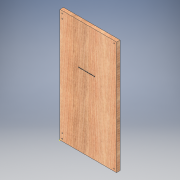
# Autodesk Inventor part: Middle Board
Saved by Autodesk Inventor 2018 (Build 220112000, 112)
## iProperties
Created: 2018-12-30
Part Number: Middle Board
Material: Generic
Document SubType Name: Modeling
Designer: maste
Density: 1 g/cm^3
Appearance: Default
Author: maste
Autodesk Inventor part; units mm, degrees
(part 1 of 2)
ref_plane "YZ Plane" through (0, 0, 0) normal (1, 0, 0) x (0, 1, 0)
ref_plane "XZ Plane" through (0, 0, 0) normal (0, 1, 0) x (-1, 0, 0)
ref_plane "XY Plane" through (0, 0, 0) normal (0, 0, 1) x (1, 0, 0)
sketch "Sketch1" plane through (0, 0, 0) normal (0, 0, 1) x (1, 0, 0)
  line L0 (0, 0) -> (304.8, 0)
  line L1 (304.8, 0) -> (304.8, 609.6)
  line L2 (304.8, 609.6) -> (0, 609.6)
  line L3 (0, 609.6) -> (0, 0)
  dimension "d0" = 304.8
  dimension "d1" = 609.6
  constraints: 8 end point, 2 parallel, 1 horizontal, 1 perpendicular
  measures "d0" distance of L2.end L1.end
  measures "d1" distance of L1.end L0.end
extrude "Extrusion1" add sketch "Sketch1" along normal blind 19.05
sketch "Sketch2" plane through (0, 0, 19.05) normal (0, 0, 1) x (1, 0, 0)
  line L0 (0, 0) -> (12.7, 0) construction
  line L1 (12.7, 0) -> (0, 0) construction
  line L2 (0, 0) -> (304.8, 0) construction
  line L3 (12.7, 0) -> (0, 0) construction
  line L4 (0, 0) -> (0, 12.7) construction
  line L5 (0, 609.6) -> (0, 0) construction
  line L6 (0, 12.7) -> (12.7, 12.7) construction
  circle A0 centre (12.7, 12.7) radius 2.5797
  line L7 (304.8, 0) -> (304.8, 609.6) construction
  line L8 (304.8, 304.8) -> (0, 304.8) construction
  line L9 (152.4, 0) -> (152.4, 609.6) construction
  line L10 (304.8, 609.6) -> (0, 609.6) construction
  circle A1 centre (12.7, 596.9) radius 2.5797
  circle A2 centre (292.1, 12.7) radius 2.5797
  circle A3 centre (292.1, 596.9) radius 2.5797
  line L11 (12.7, 596.9) -> (12.7, 571.5) construction
  circle A4 centre (12.7, 571.5) radius 2.5797
  circle A5 centre (12.7, 38.1) radius 2.5797
  dimension "d4" = 12.7
  dimension "d5" = 12.7
  dimension "d6" = 12.7
  dimension "d7" = 12.7
  dimension "d8" = 5.1594
  dimension "d11" = 25.4
  constraints: 16 end point, 6 centre point, 4 midpoint, 4 symmetric about line, 2 coincident, 1 collinear, 1 perpendicular, 1 point on line, 1 vertical, 4 other
  measures "d4" distance of L0.start L0.end
  measures "d5" distance of L0.end L0.start
  measures "d6" distance of L0.end L0.start
  measures "d7" distance of L0.start L4.end
  measures "d8" diameter of A0
  measures "d11" distance of L11.start L11.end
extrude "Extrusion3" cut sketch "Sketch2" against normal blind 19.05
sketch "Sketch3" plane through (0, 0, 19.05) normal (0, 0, 1) x (1, 0, 0)
  point P0 (0, 0)
sketch "Sketch4" plane through (0, 0, 0) normal (0, 0, -1) x (-1, 0, 0)
  line L0 (-188.1338, 391.5139) -> (-89.7519, 391.5139) construction
  line L1 (-89.7519, 391.5139) -> (-89.7519, 229.2701) construction
  line L2 (-89.7519, 229.2701) -> (-188.1338, 229.2701) construction
  line L3 (-188.1338, 229.2701) -> (-188.1338, 391.5139) construction
  spline S0 degree 2 poles (-185.9379, 389.5354) (-185.9379, 388.9624) (-186.4838, 388.2856) (-186.9012, 388.2856) knots 0 0 0 1 2 2 2
  spline S1 degree 2 poles (-186.9012, 388.2856) (-187.0717, 388.2856) (-187.3335, 388.3646) (-187.4694, 388.4461) knots 0 0 0 1 2 2 2
  line L4 (-187.4694, 388.4461) -> (-187.4694, 387.4878)
  line L5 (-187.4694, 387.4878) -> (-187.8547, 387.4878)
  line L6 (-187.8547, 387.4878) -> (-187.8547, 390.6173)
  line L7 (-187.8547, 390.6173) -> (-187.4694, 390.6173)
  line L8 (-187.4694, 390.6173) -> (-187.4694, 390.3777)
  spline S2 degree 2 poles (-187.4694, 390.3777) (-187.3261, 390.5086) (-186.9753, 390.6815) (-186.7703, 390.6815) knots 0 0 0 1 2 2 2
  spline S3 degree 2 poles (-186.7703, 390.6815) (-186.3776, 390.6815) (-185.9379, 390.0591) (-185.9379, 389.5354) knots 0 0 0 1 2 2 2
  spline S4 degree 2 poles (-186.3356, 389.491) (-186.3356, 389.8837) (-186.5851, 390.3159) (-186.8642, 390.3159) knots 0 0 0 1 2 2 2
  spline S5 degree 2 poles (-186.8642, 390.3159) (-187.0272, 390.3159) (-187.3335, 390.1702) (-187.4694, 390.0566) knots 0 0 0 1 2 2 2
  line L9 (-187.4694, 390.0566) -> (-187.4694, 388.7574)
  spline S6 degree 2 poles (-187.4694, 388.7574) (-187.3187, 388.6857) (-187.1038, 388.6314) (-186.9655, 388.6314) knots 0 0 0 1 2 2 2
  spline S7 degree 2 poles (-186.9655, 388.6314) (-186.6666, 388.6314) (-186.3356, 389.071) (-186.3356, 389.491) knots 0 0 0 1 2 2 2
  line L10 (-183.7594, 388.33) -> (-184.1447, 388.33)
  line L11 (-184.1447, 388.33) -> (-184.1447, 388.582)
  spline S8 degree 2 poles (-184.1447, 388.582) (-184.3226, 388.4264) (-184.6412, 388.2658) (-184.8388, 388.2658) knots 0 0 0 1 2 2 2
  spline S9 degree 2 poles (-184.8388, 388.2658) (-184.987, 388.2658) (-185.2513, 388.3646) (-185.3476, 388.4708) knots 0 0 0 1 2 2 2
  spline S10 degree 2 poles (-185.3476, 388.4708) (-185.4464, 388.577) (-185.5551, 388.9006) (-185.5551, 389.1328) knots 0 0 0 1 2 2 2
  line L12 (-185.5551, 389.1328) -> (-185.5551, 390.6173)
  line L13 (-185.5551, 390.6173) -> (-185.1698, 390.6173)
  line L14 (-185.1698, 390.6173) -> (-185.1698, 389.3131)
  spline S11 degree 2 poles (-185.1698, 389.3131) (-185.1698, 389.1303) (-185.1426, 388.8907) (-185.0957, 388.8018) knots 0 0 0 1 2 2 2
  spline S12 degree 2 poles (-185.0957, 388.8018) (-185.0487, 388.7129) (-184.8882, 388.6314) (-184.7375, 388.6314) knots 0 0 0 1 2 2 2
  spline S13 degree 2 poles (-184.7375, 388.6314) (-184.5967, 388.6314) (-184.2781, 388.7919) (-184.1447, 388.908) knots 0 0 0 1 2 2 2
  line L15 (-184.1447, 388.908) -> (-184.1447, 390.6173)
  line L16 (-184.1447, 390.6173) -> (-183.7594, 390.6173)
  line L17 (-183.7594, 390.6173) -> (-183.7594, 388.33)
  spline S14 degree 2 poles (-182.5096, 388.2856) (-182.8233, 388.2856) (-183.1765, 388.6437) (-183.1765, 389.0315) knots 0 0 0 1 2 2 2
  line L18 (-183.1765, 389.0315) -> (-183.1765, 390.2986)
  line L19 (-183.1765, 390.2986) -> (-183.4358, 390.2986)
  line L20 (-183.4358, 390.2986) -> (-183.4358, 390.6173)
  line L21 (-183.4358, 390.6173) -> (-183.1765, 390.6173)
  line L22 (-183.1765, 390.6173) -> (-183.1765, 391.2743)
  line L23 (-183.1765, 391.2743) -> (-182.7911, 391.2743)
  line L24 (-182.7911, 391.2743) -> (-182.7911, 390.6173)
  line L25 (-182.7911, 390.6173) -> (-182.0822, 390.6173)
  line L26 (-182.0822, 390.6173) -> (-182.0822, 390.2986)
  line L27 (-182.0822, 390.2986) -> (-182.7911, 390.2986)
  line L28 (-182.7911, 390.2986) -> (-182.7911, 389.2094)
  spline S15 degree 2 poles (-182.7911, 389.2094) (-182.7911, 389.0365) (-182.7788, 388.8463) (-182.7368, 388.7648) knots 0 0 0 1 2 2 2
  spline S16 degree 2 poles (-182.7368, 388.7648) (-182.7022, 388.6931) (-182.5466, 388.6215) (-182.4132, 388.6215) knots 0 0 0 1 2 2 2
  spline S17 degree 2 poles (-182.4132, 388.6215) (-182.3194, 388.6215) (-182.144, 388.6783) (-182.1045, 388.6956) knots 0 0 0 1 2 2 2
  line L29 (-182.1045, 388.6956) -> (-182.0822, 388.6956)
  line L30 (-182.0822, 388.6956) -> (-182.0822, 388.3498)
  spline S18 degree 2 poles (-182.0822, 388.3498) (-182.1909, 388.3202) (-182.4132, 388.2856) (-182.5096, 388.2856) knots 0 0 0 1 2 2 2
  spline S19 degree 2 poles (-179.8716, 388.2757) (-180.1013, 388.2757) (-180.499, 388.3992) (-180.6299, 388.4684) knots 0 0 0 1 2 2 2
  line L31 (-180.6299, 388.4684) -> (-180.6299, 388.9006)
  line L32 (-180.6299, 388.9006) -> (-180.6101, 388.9006)
  spline S20 degree 2 poles (-180.6101, 388.9006) (-180.5607, 388.8611) (-180.4273, 388.7672) (-180.3162, 388.7154) knots 0 0 0 1 2 2 2
  spline S21 degree 2 poles (-180.3162, 388.7154) (-180.2199, 388.6684) (-179.9827, 388.5993) (-179.8568, 388.5993) knots 0 0 0 1 2 2 2
  spline S22 degree 2 poles (-179.8568, 388.5993) (-179.7654, 388.5993) (-179.5554, 388.6413) (-179.506, 388.6758) knots 0 0 0 1 2 2 2
  spline S23 degree 2 poles (-179.506, 388.6758) (-179.4344, 388.7228) (-179.3702, 388.829) (-179.3702, 388.9377) knots 0 0 0 1 2 2 2
  spline S24 degree 2 poles (-179.3702, 388.9377) (-179.3702, 389.0735) (-179.5184, 389.2143) (-179.7086, 389.2612) knots 0 0 0 1 2 2 2
  spline S25 degree 2 poles (-179.7086, 389.2612) (-179.7827, 389.2785) (-180.0198, 389.3279) (-180.1211, 389.3551) knots 0 0 0 1 2 2 2
  spline S26 degree 2 poles (-180.1211, 389.3551) (-180.3829, 389.4317) (-180.62, 389.7478) (-180.62, 389.9726) knots 0 0 0 1 2 2 2
  spline S27 degree 2 poles (-180.62, 389.9726) (-180.62, 390.2838) (-180.1532, 390.6716) (-179.7678, 390.6716) knots 0 0 0 1 2 2 2
  spline S28 degree 2 poles (-179.7678, 390.6716) (-179.5777, 390.6716) (-179.1923, 390.5778) (-179.0614, 390.5061) knots 0 0 0 1 2 2 2
  line L33 (-179.0614, 390.5061) -> (-179.0614, 390.0936)
  line L34 (-179.0614, 390.0936) -> (-179.0812, 390.0936)
  spline S29 degree 2 poles (-179.0812, 390.0936) (-179.2294, 390.2122) (-179.59, 390.348) (-179.7753, 390.348) knots 0 0 0 1 2 2 2
  spline S30 degree 2 poles (-179.7753, 390.348) (-179.9654, 390.348) (-180.2273, 390.1875) (-180.2273, 390.0269) knots 0 0 0 1 2 2 2
  spline S31 degree 2 poles (-180.2273, 390.0269) (-180.2273, 389.8812) (-180.0717, 389.7404) (-179.8988, 389.696) knots 0 0 0 1 2 2 2
  spline S32 degree 2 poles (-179.8988, 389.696) (-179.8148, 389.6737) (-179.6024, 389.6293) (-179.4863, 389.6021) knots 0 0 0 1 2 2 2
  spline S33 degree 2 poles (-179.4863, 389.6021) (-179.2343, 389.5379) (-178.9774, 389.2439) (-178.9774, 388.9895) knots 0 0 0 1 2 2 2
  spline S34 degree 2 poles (-178.9774, 388.9895) (-178.9774, 388.8413) (-179.0935, 388.5795) (-179.2071, 388.4832) knots 0 0 0 1 2 2 2
  spline S35 degree 2 poles (-179.2071, 388.4832) (-179.3282, 388.3819) (-179.6369, 388.2757) (-179.8716, 388.2757) knots 0 0 0 1 2 2 2
  spline S36 degree 2 poles (-176.7396, 389.4737) (-176.7396, 388.8957) (-177.2954, 388.2658) (-177.7597, 388.2658) knots 0 0 0 1 2 2 2
  spline S37 degree 2 poles (-177.7597, 388.2658) (-178.2364, 388.2658) (-178.7823, 388.9154) (-178.7823, 389.4737) knots 0 0 0 1 2 2 2
  spline S38 degree 2 poles (-178.7823, 389.4737) (-178.7823, 390.0467) (-178.2191, 390.6815) (-177.7597, 390.6815) knots 0 0 0 1 2 2 2
  spline S39 degree 2 poles (-177.7597, 390.6815) (-177.2954, 390.6815) (-176.7396, 390.0492) (-176.7396, 389.4737) knots 0 0 0 1 2 2 2
  spline S40 degree 2 poles (-177.1373, 389.4737) (-177.1373, 389.9183) (-177.4608, 390.3505) (-177.7597, 390.3505) knots 0 0 0 1 2 2 2
  spline S41 degree 2 poles (-177.7597, 390.3505) (-178.0586, 390.3505) (-178.3846, 389.9183) (-178.3846, 389.4737) knots 0 0 0 1 2 2 2
  spline S42 degree 2 poles (-178.3846, 389.4737) (-178.3846, 389.0414) (-178.0586, 388.5968) (-177.7597, 388.5968) knots 0 0 0 1 2 2 2
  spline S43 degree 2 poles (-177.7597, 388.5968) (-177.4633, 388.5968) (-177.1373, 389.034) (-177.1373, 389.4737) knots 0 0 0 1 2 2 2
  line L35 (-173.7509, 388.33) -> (-173.7509, 389.654)
  spline S44 degree 2 poles (-173.7509, 389.654) (-173.7509, 389.8121) (-173.7756, 390.0813) (-173.8151, 390.1554) knots 0 0 0 1 2 2 2
  spline S45 degree 2 poles (-173.8151, 390.1554) (-173.8546, 390.2369) (-174.0053, 390.3159) (-174.1362, 390.3159) knots 0 0 0 1 2 2 2
  spline S46 degree 2 poles (-174.1362, 390.3159) (-174.2548, 390.3159) (-174.5265, 390.1702) (-174.6697, 390.0319) knots 0 0 0 1 2 2 2
  spline S47 degree 2 poles (-174.6697, 390.0319) (-174.6673, 389.9973) (-174.6623, 389.901) (-174.6623, 389.8368) knots 0 0 0 1 2 2 2
  line L36 (-174.6623, 389.8368) -> (-174.6623, 388.33)
  line L37 (-174.6623, 388.33) -> (-175.0476, 388.33)
  line L38 (-175.0476, 388.33) -> (-175.0476, 389.654)
  spline S48 degree 2 poles (-175.0476, 389.654) (-175.0476, 389.8121) (-175.0723, 390.0813) (-175.1119, 390.1554) knots 0 0 0 1 2 2 2
  spline S49 degree 2 poles (-175.1119, 390.1554) (-175.1514, 390.2369) (-175.3021, 390.3159) (-175.433, 390.3159) knots 0 0 0 1 2 2 2
  spline S50 degree 2 poles (-175.433, 390.3159) (-175.5565, 390.3159) (-175.8306, 390.1603) (-175.9591, 390.0393) knots 0 0 0 1 2 2 2
  line L39 (-175.9591, 390.0393) -> (-175.9591, 388.33)
  line L40 (-175.9591, 388.33) -> (-176.3444, 388.33)
  line L41 (-176.3444, 388.33) -> (-176.3444, 390.6173)
  line L42 (-176.3444, 390.6173) -> (-175.9591, 390.6173)
  line L43 (-175.9591, 390.6173) -> (-175.9591, 390.3653)
  spline S51 degree 2 poles (-175.9591, 390.3653) (-175.8084, 390.516) (-175.512, 390.6815) (-175.3342, 390.6815) knots 0 0 0 1 2 2 2
  spline S52 degree 2 poles (-175.3342, 390.6815) (-175.1316, 390.6815) (-174.8179, 390.4962) (-174.7364, 390.2863) knots 0 0 0 1 2 2 2
  spline S53 degree 2 poles (-174.7364, 390.2863) (-174.561, 390.4814) (-174.2301, 390.6815) (-174.0374, 390.6815) knots 0 0 0 1 2 2 2
  spline S54 degree 2 poles (-174.0374, 390.6815) (-173.8892, 390.6815) (-173.6471, 390.5901) (-173.5582, 390.4864) knots 0 0 0 1 2 2 2
  spline S55 degree 2 poles (-173.5582, 390.4864) (-173.4668, 390.3826) (-173.3656, 390.0714) (-173.3656, 389.8368) knots 0 0 0 1 2 2 2
  line L44 (-173.3656, 389.8368) -> (-173.3656, 388.33)
  line L45 (-173.3656, 388.33) -> (-173.7509, 388.33)
  spline S56 degree 2 poles (-171.8317, 388.2782) (-172.38, 388.2782) (-172.9827, 388.8932) (-172.9827, 389.4613) knots 0 0 0 1 2 2 2
  spline S57 degree 2 poles (-172.9827, 389.4613) (-172.9827, 390.0195) (-172.3973, 390.6815) (-171.9255, 390.6815) knots 0 0 0 1 2 2 2
  spline S58 degree 2 poles (-171.9255, 390.6815) (-171.7131, 390.6815) (-171.3846, 390.558) (-171.2636, 390.4271) knots 0 0 0 1 2 2 2
  spline S59 degree 2 poles (-171.2636, 390.4271) (-171.1401, 390.2962) (-171.0092, 389.9183) (-171.0092, 389.6441) knots 0 0 0 1 2 2 2
  line L46 (-171.0092, 389.6441) -> (-171.0092, 389.4341)
  line L47 (-171.0092, 389.4341) -> (-172.5924, 389.4341)
  spline S60 degree 2 poles (-172.5924, 389.4341) (-172.5924, 389.0365) (-172.1923, 388.6141) (-171.8366, 388.6141) knots 0 0 0 1 2 2 2
  spline S61 degree 2 poles (-171.8366, 388.6141) (-171.7106, 388.6141) (-171.4661, 388.6709) (-171.3673, 388.7154) knots 0 0 0 1 2 2 2
  spline S62 degree 2 poles (-171.3673, 388.7154) (-171.2636, 388.7648) (-171.1203, 388.8512) (-171.0734, 388.8907) knots 0 0 0 1 2 2 2
  line L48 (-171.0734, 388.8907) -> (-171.0512, 388.8907)
  line L49 (-171.0512, 388.8907) -> (-171.0512, 388.4708)
  spline S63 degree 2 poles (-171.0512, 388.4708) (-171.1178, 388.4437) (-171.3204, 388.3646) (-171.3994, 388.3424) knots 0 0 0 1 2 2 2
  spline S64 degree 2 poles (-171.3994, 388.3424) (-171.5106, 388.3103) (-171.6934, 388.2782) (-171.8317, 388.2782) knots 0 0 0 1 2 2 2
  spline S65 degree 2 poles (-171.3846, 389.7281) (-171.3895, 389.8837) (-171.4538, 390.1109) (-171.5155, 390.1875) knots 0 0 0 1 2 2 2
  spline S66 degree 2 poles (-171.5155, 390.1875) (-171.5822, 390.2739) (-171.7922, 390.3653) (-171.9478, 390.3653) knots 0 0 0 1 2 2 2
  spline S67 degree 2 poles (-171.9478, 390.3653) (-172.1009, 390.3653) (-172.3158, 390.2739) (-172.4047, 390.185) knots 0 0 0 1 2 2 2
  spline S68 degree 2 poles (-172.4047, 390.185) (-172.4912, 390.0936) (-172.5801, 389.8738) (-172.5924, 389.7281) knots 0 0 0 1 2 2 2
  line L50 (-172.5924, 389.7281) -> (-171.3846, 389.7281)
  line L51 (-168.9171, 388.33) -> (-169.3024, 388.33)
  line L52 (-169.3024, 388.33) -> (-169.3024, 391.5139)
  line L53 (-169.3024, 391.5139) -> (-168.9171, 391.5139)
  line L54 (-168.9171, 391.5139) -> (-168.9171, 388.33)
  spline S69 degree 2 poles (-167.0769, 388.5721) (-167.1238, 388.5375) (-167.2819, 388.414) (-167.356, 388.377) knots 0 0 0 1 2 2 2
  spline S70 degree 2 poles (-167.356, 388.377) (-167.4573, 388.3226) (-167.6475, 388.2658) (-167.8204, 388.2658) knots 0 0 0 1 2 2 2
  spline S71 degree 2 poles (-167.8204, 388.2658) (-167.9612, 388.2658) (-168.2156, 388.372) (-168.3119, 388.4684) knots 0 0 0 1 2 2 2
  spline S72 degree 2 poles (-168.3119, 388.4684) (-168.4033, 388.5622) (-168.5144, 388.8389) (-168.5144, 388.992) knots 0 0 0 1 2 2 2
  spline S73 degree 2 poles (-168.5144, 388.992) (-168.5144, 389.2291) (-168.3144, 389.5651) (-168.097, 389.6614) knots 0 0 0 1 2 2 2
  spline S74 degree 2 poles (-168.097, 389.6614) (-167.9044, 389.7503) (-167.3807, 389.817) (-167.0769, 389.8343) knots 0 0 0 1 2 2 2
  line L55 (-167.0769, 389.8343) -> (-167.0769, 389.9084)
  spline S75 degree 2 poles (-167.0769, 389.9084) (-167.0769, 390.0418) (-167.1584, 390.2073) (-167.2325, 390.2542) knots 0 0 0 1 2 2 2
  spline S76 degree 2 poles (-167.2325, 390.2542) (-167.3066, 390.3011) (-167.519, 390.3308) (-167.6327, 390.3308) knots 0 0 0 1 2 2 2
  spline S77 degree 2 poles (-167.6327, 390.3308) (-167.766, 390.3308) (-168.1267, 390.2517) (-168.307, 390.1751) knots 0 0 0 1 2 2 2
  line L56 (-168.307, 390.1751) -> (-168.3292, 390.1751)
  line L57 (-168.3292, 390.1751) -> (-168.3292, 390.5679)
  spline S78 degree 2 poles (-168.3292, 390.5679) (-168.223, 390.5975) (-167.8253, 390.6716) (-167.6302, 390.6716) knots 0 0 0 1 2 2 2
  spline S79 degree 2 poles (-167.6302, 390.6716) (-167.3931, 390.6716) (-167.0695, 390.5975) (-166.941, 390.5012) knots 0 0 0 1 2 2 2
  spline S80 degree 2 poles (-166.941, 390.5012) (-166.8151, 390.4073) (-166.6916, 390.1085) (-166.6916, 389.8936) knots 0 0 0 1 2 2 2
  line L58 (-166.6916, 389.8936) -> (-166.6916, 388.33)
  line L59 (-166.6916, 388.33) -> (-167.0769, 388.33)
  line L60 (-167.0769, 388.33) -> (-167.0769, 388.5721)
  line L61 (-167.0769, 388.8932) -> (-167.0769, 389.528)
  spline S81 degree 2 poles (-167.0769, 389.528) (-167.2152, 389.5157) (-167.6327, 389.4737) (-167.7636, 389.4341) knots 0 0 0 1 2 2 2
  spline S82 degree 2 poles (-167.7636, 389.4341) (-167.9167, 389.3872) (-168.1168, 389.1921) (-168.1168, 389.0192) knots 0 0 0 1 2 2 2
  spline S83 degree 2 poles (-168.1168, 389.0192) (-168.1168, 388.8216) (-167.8945, 388.6215) (-167.6821, 388.6215) knots 0 0 0 1 2 2 2
  spline S84 degree 2 poles (-167.6821, 388.6215) (-167.5017, 388.6215) (-167.2053, 388.7771) (-167.0769, 388.8932) knots 0 0 0 1 2 2 2
  spline S85 degree 2 poles (-164.2339, 389.5354) (-164.2339, 388.9624) (-164.7798, 388.2856) (-165.1972, 388.2856) knots 0 0 0 1 2 2 2
  spline S86 degree 2 poles (-165.1972, 388.2856) (-165.3676, 388.2856) (-165.6295, 388.3646) (-165.7653, 388.4461) knots 0 0 0 1 2 2 2
  line L62 (-165.7653, 388.4461) -> (-165.7653, 387.4878)
  line L63 (-165.7653, 387.4878) -> (-166.1506, 387.4878)
  line L64 (-166.1506, 387.4878) -> (-166.1506, 390.6173)
  line L65 (-166.1506, 390.6173) -> (-165.7653, 390.6173)
  line L66 (-165.7653, 390.6173) -> (-165.7653, 390.3777)
  spline S87 degree 2 poles (-165.7653, 390.3777) (-165.6221, 390.5086) (-165.2713, 390.6815) (-165.0663, 390.6815) knots 0 0 0 1 2 2 2
  spline S88 degree 2 poles (-165.0663, 390.6815) (-164.6736, 390.6815) (-164.2339, 390.0591) (-164.2339, 389.5354) knots 0 0 0 1 2 2 2
  spline S89 degree 2 poles (-164.6316, 389.491) (-164.6316, 389.8837) (-164.8811, 390.3159) (-165.1602, 390.3159) knots 0 0 0 1 2 2 2
  spline S90 degree 2 poles (-165.1602, 390.3159) (-165.3232, 390.3159) (-165.6295, 390.1702) (-165.7653, 390.0566) knots 0 0 0 1 2 2 2
  line L67 (-165.7653, 390.0566) -> (-165.7653, 388.7574)
  spline S91 degree 2 poles (-165.7653, 388.7574) (-165.6146, 388.6857) (-165.3998, 388.6314) (-165.2614, 388.6314) knots 0 0 0 1 2 2 2
  spline S92 degree 2 poles (-165.2614, 388.6314) (-164.9626, 388.6314) (-164.6316, 389.071) (-164.6316, 389.491) knots 0 0 0 1 2 2 2
  spline S93 degree 2 poles (-163.1422, 388.2856) (-163.4559, 388.2856) (-163.8091, 388.6437) (-163.8091, 389.0315) knots 0 0 0 1 2 2 2
  line L68 (-163.8091, 389.0315) -> (-163.8091, 390.2986)
  line L69 (-163.8091, 390.2986) -> (-164.0684, 390.2986)
  line L70 (-164.0684, 390.2986) -> (-164.0684, 390.6173)
  line L71 (-164.0684, 390.6173) -> (-163.8091, 390.6173)
  line L72 (-163.8091, 390.6173) -> (-163.8091, 391.2743)
  line L73 (-163.8091, 391.2743) -> (-163.4237, 391.2743)
  line L74 (-163.4237, 391.2743) -> (-163.4237, 390.6173)
  line L75 (-163.4237, 390.6173) -> (-162.7149, 390.6173)
  line L76 (-162.7149, 390.6173) -> (-162.7149, 390.2986)
  line L77 (-162.7149, 390.2986) -> (-163.4237, 390.2986)
  line L78 (-163.4237, 390.2986) -> (-163.4237, 389.2094)
  spline S94 degree 2 poles (-163.4237, 389.2094) (-163.4237, 389.0365) (-163.4114, 388.8463) (-163.3694, 388.7648) knots 0 0 0 1 2 2 2
  spline S95 degree 2 poles (-163.3694, 388.7648) (-163.3348, 388.6931) (-163.1792, 388.6215) (-163.0458, 388.6215) knots 0 0 0 1 2 2 2
  spline S96 degree 2 poles (-163.0458, 388.6215) (-162.952, 388.6215) (-162.7766, 388.6783) (-162.7371, 388.6956) knots 0 0 0 1 2 2 2
  line L79 (-162.7371, 388.6956) -> (-162.7149, 388.6956)
  line L80 (-162.7149, 388.6956) -> (-162.7149, 388.3498)
  spline S97 degree 2 poles (-162.7149, 388.3498) (-162.8235, 388.3202) (-163.0458, 388.2856) (-163.1422, 388.2856) knots 0 0 0 1 2 2 2
  spline S98 degree 2 poles (-160.5511, 389.4737) (-160.5511, 388.8957) (-161.1069, 388.2658) (-161.5712, 388.2658) knots 0 0 0 1 2 2 2
  spline S99 degree 2 poles (-161.5712, 388.2658) (-162.0479, 388.2658) (-162.5938, 388.9154) (-162.5938, 389.4737) knots 0 0 0 1 2 2 2
  spline S100 degree 2 poles (-162.5938, 389.4737) (-162.5938, 390.0467) (-162.0307, 390.6815) (-161.5712, 390.6815) knots 0 0 0 1 2 2 2
  spline S101 degree 2 poles (-161.5712, 390.6815) (-161.1069, 390.6815) (-160.5511, 390.0492) (-160.5511, 389.4737) knots 0 0 0 1 2 2 2
  spline S102 degree 2 poles (-160.9488, 389.4737) (-160.9488, 389.9183) (-161.2724, 390.3505) (-161.5712, 390.3505) knots 0 0 0 1 2 2 2
  spline S103 degree 2 poles (-161.5712, 390.3505) (-161.8701, 390.3505) (-162.1961, 389.9183) (-162.1961, 389.4737) knots 0 0 0 1 2 2 2
  spline S104 degree 2 poles (-162.1961, 389.4737) (-162.1961, 389.0414) (-161.8701, 388.5968) (-161.5712, 388.5968) knots 0 0 0 1 2 2 2
  spline S105 degree 2 poles (-161.5712, 388.5968) (-161.2748, 388.5968) (-160.9488, 389.034) (-160.9488, 389.4737) knots 0 0 0 1 2 2 2
  spline S106 degree 2 poles (-158.2392, 389.5354) (-158.2392, 388.9624) (-158.7851, 388.2856) (-159.2025, 388.2856) knots 0 0 0 1 2 2 2
  spline S107 degree 2 poles (-159.2025, 388.2856) (-159.3729, 388.2856) (-159.6347, 388.3646) (-159.7706, 388.4461) knots 0 0 0 1 2 2 2
  line L81 (-159.7706, 388.4461) -> (-159.7706, 387.4878)
  line L82 (-159.7706, 387.4878) -> (-160.1559, 387.4878)
  line L83 (-160.1559, 387.4878) -> (-160.1559, 390.6173)
  line L84 (-160.1559, 390.6173) -> (-159.7706, 390.6173)
  line L85 (-159.7706, 390.6173) -> (-159.7706, 390.3777)
  spline S108 degree 2 poles (-159.7706, 390.3777) (-159.6273, 390.5086) (-159.2766, 390.6815) (-159.0716, 390.6815) knots 0 0 0 1 2 2 2
  spline S109 degree 2 poles (-159.0716, 390.6815) (-158.6788, 390.6815) (-158.2392, 390.0591) (-158.2392, 389.5354) knots 0 0 0 1 2 2 2
  spline S110 degree 2 poles (-158.6369, 389.491) (-158.6369, 389.8837) (-158.8863, 390.3159) (-159.1654, 390.3159) knots 0 0 0 1 2 2 2
  spline S111 degree 2 poles (-159.1654, 390.3159) (-159.3285, 390.3159) (-159.6347, 390.1702) (-159.7706, 390.0566) knots 0 0 0 1 2 2 2
  line L86 (-159.7706, 390.0566) -> (-159.7706, 388.7574)
  spline S112 degree 2 poles (-159.7706, 388.7574) (-159.6199, 388.6857) (-159.405, 388.6314) (-159.2667, 388.6314) knots 0 0 0 1 2 2 2
  spline S113 degree 2 poles (-159.2667, 388.6314) (-158.9678, 388.6314) (-158.6369, 389.071) (-158.6369, 389.491) knots 0 0 0 1 2 2 2
  spline S114 degree 2 poles (-157.2215, 388.2757) (-157.4512, 388.2757) (-157.8489, 388.3992) (-157.9798, 388.4684) knots 0 0 0 1 2 2 2
  line L87 (-157.9798, 388.4684) -> (-157.9798, 388.9006)
  line L88 (-157.9798, 388.9006) -> (-157.9601, 388.9006)
  spline S115 degree 2 poles (-157.9601, 388.9006) (-157.9107, 388.8611) (-157.7773, 388.7672) (-157.6661, 388.7154) knots 0 0 0 1 2 2 2
  spline S116 degree 2 poles (-157.6661, 388.7154) (-157.5698, 388.6684) (-157.3327, 388.5993) (-157.2067, 388.5993) knots 0 0 0 1 2 2 2
  spline S117 degree 2 poles (-157.2067, 388.5993) (-157.1153, 388.5993) (-156.9054, 388.6413) (-156.856, 388.6758) knots 0 0 0 1 2 2 2
  spline S118 degree 2 poles (-156.856, 388.6758) (-156.7843, 388.7228) (-156.7201, 388.829) (-156.7201, 388.9377) knots 0 0 0 1 2 2 2
  spline S119 degree 2 poles (-156.7201, 388.9377) (-156.7201, 389.0735) (-156.8683, 389.2143) (-157.0585, 389.2612) knots 0 0 0 1 2 2 2
  spline S120 degree 2 poles (-157.0585, 389.2612) (-157.1326, 389.2785) (-157.3697, 389.3279) (-157.471, 389.3551) knots 0 0 0 1 2 2 2
  spline S121 degree 2 poles (-157.471, 389.3551) (-157.7328, 389.4317) (-157.9699, 389.7478) (-157.9699, 389.9726) knots 0 0 0 1 2 2 2
  spline S122 degree 2 poles (-157.9699, 389.9726) (-157.9699, 390.2838) (-157.5031, 390.6716) (-157.1178, 390.6716) knots 0 0 0 1 2 2 2
  spline S123 degree 2 poles (-157.1178, 390.6716) (-156.9276, 390.6716) (-156.5423, 390.5778) (-156.4114, 390.5061) knots 0 0 0 1 2 2 2
  line L89 (-156.4114, 390.5061) -> (-156.4114, 390.0936)
  line L90 (-156.4114, 390.0936) -> (-156.4311, 390.0936)
  spline S124 degree 2 poles (-156.4311, 390.0936) (-156.5793, 390.2122) (-156.94, 390.348) (-157.1252, 390.348) knots 0 0 0 1 2 2 2
  spline S125 degree 2 poles (-157.1252, 390.348) (-157.3154, 390.348) (-157.5772, 390.1875) (-157.5772, 390.0269) knots 0 0 0 1 2 2 2
  spline S126 degree 2 poles (-157.5772, 390.0269) (-157.5772, 389.8812) (-157.4216, 389.7404) (-157.2487, 389.696) knots 0 0 0 1 2 2 2
  spline S127 degree 2 poles (-157.2487, 389.696) (-157.1647, 389.6737) (-156.9523, 389.6293) (-156.8362, 389.6021) knots 0 0 0 1 2 2 2
  spline S128 degree 2 poles (-156.8362, 389.6021) (-156.5843, 389.5379) (-156.3274, 389.2439) (-156.3274, 388.9895) knots 0 0 0 1 2 2 2
  spline S129 degree 2 poles (-156.3274, 388.9895) (-156.3274, 388.8413) (-156.4435, 388.5795) (-156.5571, 388.4832) knots 0 0 0 1 2 2 2
  spline S130 degree 2 poles (-156.5571, 388.4832) (-156.6781, 388.3819) (-156.9869, 388.2757) (-157.2215, 388.2757) knots 0 0 0 1 2 2 2
  spline S131 degree 2 poles (-153.3856, 388.5721) (-153.4325, 388.5375) (-153.5906, 388.414) (-153.6647, 388.377) knots 0 0 0 1 2 2 2
  spline S132 degree 2 poles (-153.6647, 388.377) (-153.766, 388.3226) (-153.9562, 388.2658) (-154.1291, 388.2658) knots 0 0 0 1 2 2 2
  spline S133 degree 2 poles (-154.1291, 388.2658) (-154.2699, 388.2658) (-154.5243, 388.372) (-154.6206, 388.4684) knots 0 0 0 1 2 2 2
  spline S134 degree 2 poles (-154.6206, 388.4684) (-154.712, 388.5622) (-154.8231, 388.8389) (-154.8231, 388.992) knots 0 0 0 1 2 2 2
  spline S135 degree 2 poles (-154.8231, 388.992) (-154.8231, 389.2291) (-154.6231, 389.5651) (-154.4057, 389.6614) knots 0 0 0 1 2 2 2
  spline S136 degree 2 poles (-154.4057, 389.6614) (-154.2131, 389.7503) (-153.6894, 389.817) (-153.3856, 389.8343) knots 0 0 0 1 2 2 2
  line L91 (-153.3856, 389.8343) -> (-153.3856, 389.9084)
  spline S137 degree 2 poles (-153.3856, 389.9084) (-153.3856, 390.0418) (-153.4671, 390.2073) (-153.5412, 390.2542) knots 0 0 0 1 2 2 2
  spline S138 degree 2 poles (-153.5412, 390.2542) (-153.6153, 390.3011) (-153.8277, 390.3308) (-153.9414, 390.3308) knots 0 0 0 1 2 2 2
  spline S139 degree 2 poles (-153.9414, 390.3308) (-154.0747, 390.3308) (-154.4354, 390.2517) (-154.6157, 390.1751) knots 0 0 0 1 2 2 2
  line L92 (-154.6157, 390.1751) -> (-154.6379, 390.1751)
  line L93 (-154.6379, 390.1751) -> (-154.6379, 390.5679)
  spline S140 degree 2 poles (-154.6379, 390.5679) (-154.5317, 390.5975) (-154.134, 390.6716) (-153.9389, 390.6716) knots 0 0 0 1 2 2 2
  spline S141 degree 2 poles (-153.9389, 390.6716) (-153.7018, 390.6716) (-153.3782, 390.5975) (-153.2497, 390.5012) knots 0 0 0 1 2 2 2
  spline S142 degree 2 poles (-153.2497, 390.5012) (-153.1238, 390.4073) (-153.0003, 390.1085) (-153.0003, 389.8936) knots 0 0 0 1 2 2 2
  line L94 (-153.0003, 389.8936) -> (-153.0003, 388.33)
  line L95 (-153.0003, 388.33) -> (-153.3856, 388.33)
  line L96 (-153.3856, 388.33) -> (-153.3856, 388.5721)
  line L97 (-153.3856, 388.8932) -> (-153.3856, 389.528)
  spline S143 degree 2 poles (-153.3856, 389.528) (-153.5239, 389.5157) (-153.9414, 389.4737) (-154.0723, 389.4341) knots 0 0 0 1 2 2 2
  spline S144 degree 2 poles (-154.0723, 389.4341) (-154.2254, 389.3872) (-154.4255, 389.1921) (-154.4255, 389.0192) knots 0 0 0 1 2 2 2
  spline S145 degree 2 poles (-154.4255, 389.0192) (-154.4255, 388.8216) (-154.2032, 388.6215) (-153.9908, 388.6215) knots 0 0 0 1 2 2 2
  spline S146 degree 2 poles (-153.9908, 388.6215) (-153.8104, 388.6215) (-153.514, 388.7771) (-153.3856, 388.8932) knots 0 0 0 1 2 2 2
  line L98 (-150.6636, 388.33) -> (-151.049, 388.33)
  line L99 (-151.049, 388.33) -> (-151.049, 389.6342)
  spline S147 degree 2 poles (-151.049, 389.6342) (-151.049, 389.7923) (-151.0786, 390.064) (-151.1231, 390.1455) knots 0 0 0 1 2 2 2
  spline S148 degree 2 poles (-151.1231, 390.1455) (-151.17, 390.232) (-151.338, 390.3159) (-151.4812, 390.3159) knots 0 0 0 1 2 2 2
  spline S149 degree 2 poles (-151.4812, 390.3159) (-151.6245, 390.3159) (-151.9283, 390.1628) (-152.074, 390.0393) knots 0 0 0 1 2 2 2
  line L100 (-152.074, 390.0393) -> (-152.074, 388.33)
  line L101 (-152.074, 388.33) -> (-152.4593, 388.33)
  line L102 (-152.4593, 388.33) -> (-152.4593, 390.6173)
  line L103 (-152.4593, 390.6173) -> (-152.074, 390.6173)
  line L104 (-152.074, 390.6173) -> (-152.074, 390.3629)
  spline S150 degree 2 poles (-152.074, 390.3629) (-151.9011, 390.5185) (-151.5677, 390.6815) (-151.3799, 390.6815) knots 0 0 0 1 2 2 2
  spline S151 degree 2 poles (-151.3799, 390.6815) (-151.044, 390.6815) (-150.6636, 390.2369) (-150.6636, 389.8145) knots 0 0 0 1 2 2 2
  line L105 (-150.6636, 389.8145) -> (-150.6636, 388.33)
  line L106 (-148.3641, 388.33) -> (-148.7494, 388.33)
  line L107 (-148.7494, 388.33) -> (-148.7494, 388.5622)
  spline S152 degree 2 poles (-148.7494, 388.5622) (-148.8383, 388.4881) (-148.9692, 388.3893) (-149.0581, 388.3473) knots 0 0 0 1 2 2 2
  spline S153 degree 2 poles (-149.0581, 388.3473) (-149.1396, 388.3078) (-149.315, 388.2658) (-149.4311, 388.2658) knots 0 0 0 1 2 2 2
  spline S154 degree 2 poles (-149.4311, 388.2658) (-149.6188, 388.2658) (-149.935, 388.4214) (-150.0461, 388.5721) knots 0 0 0 1 2 2 2
  spline S155 degree 2 poles (-150.0461, 388.5721) (-150.1573, 388.7228) (-150.2808, 389.1674) (-150.2808, 389.4564) knots 0 0 0 1 2 2 2
  spline S156 degree 2 poles (-150.2808, 389.4564) (-150.2808, 389.7577) (-150.1252, 390.1974) (-149.9893, 390.3629) knots 0 0 0 1 2 2 2
  spline S157 degree 2 poles (-149.9893, 390.3629) (-149.8634, 390.5111) (-149.5101, 390.6815) (-149.315, 390.6815) knots 0 0 0 1 2 2 2
  spline S158 degree 2 poles (-149.315, 390.6815) (-149.1446, 390.6815) (-148.8902, 390.6049) (-148.7494, 390.5259) knots 0 0 0 1 2 2 2
  line L108 (-148.7494, 390.5259) -> (-148.7494, 391.5139)
  line L109 (-148.7494, 391.5139) -> (-148.3641, 391.5139)
  line L110 (-148.3641, 391.5139) -> (-148.3641, 388.33)
  line L111 (-148.7494, 388.8858) -> (-148.7494, 390.2073)
  spline S159 degree 2 poles (-148.7494, 390.2073) (-148.8926, 390.2764) (-149.1199, 390.3283) (-149.2508, 390.3283) knots 0 0 0 1 2 2 2
  spline S160 degree 2 poles (-149.2508, 390.3283) (-149.5472, 390.3283) (-149.8831, 389.8837) (-149.8831, 389.4638) knots 0 0 0 1 2 2 2
  spline S161 degree 2 poles (-149.8831, 389.4638) (-149.8831, 389.0587) (-149.6262, 388.6314) (-149.3422, 388.6314) knots 0 0 0 1 2 2 2
  spline S162 degree 2 poles (-149.3422, 388.6314) (-149.1915, 388.6314) (-148.8852, 388.7697) (-148.7494, 388.8858) knots 0 0 0 1 2 2 2
  spline S163 degree 2 poles (-145.8743, 388.2658) (-145.8743, 387.8756) (-146.2942, 387.4655) (-146.6622, 387.4655) knots 0 0 0 1 2 2 2
  spline S164 degree 2 poles (-146.6622, 387.4655) (-146.7264, 387.4655) (-146.8845, 387.4779) (-146.9611, 387.4902) knots 0 0 0 1 2 2 2
  line L112 (-146.9611, 387.4902) -> (-146.9611, 387.836)
  line L113 (-146.9611, 387.836) -> (-146.9389, 387.836)
  spline S165 degree 2 poles (-146.9389, 387.836) (-146.8944, 387.8262) (-146.7857, 387.8064) (-146.7363, 387.8064) knots 0 0 0 1 2 2 2
  spline S166 degree 2 poles (-146.7363, 387.8064) (-146.5832, 387.8064) (-146.3831, 387.883) (-146.3362, 387.9645) knots 0 0 0 1 2 2 2
  spline S167 degree 2 poles (-146.3362, 387.9645) (-146.2892, 388.0386) (-146.2596, 388.2634) (-146.2596, 388.4239) knots 0 0 0 1 2 2 2
  line L114 (-146.2596, 388.4239) -> (-146.2596, 390.2986)
  line L115 (-146.2596, 390.2986) -> (-146.6721, 390.2986)
  line L116 (-146.6721, 390.2986) -> (-146.6721, 390.6173)
  line L117 (-146.6721, 390.6173) -> (-145.8743, 390.6173)
  line L118 (-145.8743, 390.6173) -> (-145.8743, 388.2658)
  line L119 (-145.8718, 390.9977) -> (-146.309, 390.9977)
  line L120 (-146.309, 390.9977) -> (-146.309, 391.3978)
  line L121 (-146.309, 391.3978) -> (-145.8718, 391.3978)
  line L122 (-145.8718, 391.3978) -> (-145.8718, 390.9977)
  spline S168 degree 2 poles (-143.4364, 389.4737) (-143.4364, 388.8957) (-143.9921, 388.2658) (-144.4565, 388.2658) knots 0 0 0 1 2 2 2
  spline S169 degree 2 poles (-144.4565, 388.2658) (-144.9332, 388.2658) (-145.4791, 388.9154) (-145.4791, 389.4737) knots 0 0 0 1 2 2 2
  spline S170 degree 2 poles (-145.4791, 389.4737) (-145.4791, 390.0467) (-144.9159, 390.6815) (-144.4565, 390.6815) knots 0 0 0 1 2 2 2
  spline S171 degree 2 poles (-144.4565, 390.6815) (-143.9921, 390.6815) (-143.4364, 390.0492) (-143.4364, 389.4737) knots 0 0 0 1 2 2 2
  spline S172 degree 2 poles (-143.834, 389.4737) (-143.834, 389.9183) (-144.1576, 390.3505) (-144.4565, 390.3505) knots 0 0 0 1 2 2 2
  spline S173 degree 2 poles (-144.4565, 390.3505) (-144.7554, 390.3505) (-145.0814, 389.9183) (-145.0814, 389.4737) knots 0 0 0 1 2 2 2
  spline S174 degree 2 poles (-145.0814, 389.4737) (-145.0814, 389.0414) (-144.7554, 388.5968) (-144.4565, 388.5968) knots 0 0 0 1 2 2 2
  spline S175 degree 2 poles (-144.4565, 388.5968) (-144.1601, 388.5968) (-143.834, 389.034) (-143.834, 389.4737) knots 0 0 0 1 2 2 2
  line L123 (-141.2455, 390.6173) -> (-142.4755, 387.4878)
  line L124 (-142.4755, 387.4878) -> (-142.888, 387.4878)
  line L125 (-142.888, 387.4878) -> (-142.478, 388.4412)
  line L126 (-142.478, 388.4412) -> (-143.3079, 390.6173)
  line L127 (-143.3079, 390.6173) -> (-142.893, 390.6173)
  line L128 (-142.893, 390.6173) -> (-142.2681, 388.9228)
  line L129 (-142.2681, 388.9228) -> (-141.6456, 390.6173)
  line L130 (-141.6456, 390.6173) -> (-141.2455, 390.6173)
  spline S176 degree 2 poles (-140.3365, 388.2757) (-140.5662, 388.2757) (-140.9639, 388.3992) (-141.0948, 388.4684) knots 0 0 0 1 2 2 2
  line L131 (-141.0948, 388.4684) -> (-141.0948, 388.9006)
  line L132 (-141.0948, 388.9006) -> (-141.075, 388.9006)
  spline S177 degree 2 poles (-141.075, 388.9006) (-141.0256, 388.8611) (-140.8923, 388.7672) (-140.7811, 388.7154) knots 0 0 0 1 2 2 2
  spline S178 degree 2 poles (-140.7811, 388.7154) (-140.6848, 388.6684) (-140.4477, 388.5993) (-140.3217, 388.5993) knots 0 0 0 1 2 2 2
  spline S179 degree 2 poles (-140.3217, 388.5993) (-140.2303, 388.5993) (-140.0203, 388.6413) (-139.9709, 388.6758) knots 0 0 0 1 2 2 2
  spline S180 degree 2 poles (-139.9709, 388.6758) (-139.8993, 388.7228) (-139.8351, 388.829) (-139.8351, 388.9377) knots 0 0 0 1 2 2 2
  spline S181 degree 2 poles (-139.8351, 388.9377) (-139.8351, 389.0735) (-139.9833, 389.2143) (-140.1735, 389.2612) knots 0 0 0 1 2 2 2
  spline S182 degree 2 poles (-140.1735, 389.2612) (-140.2476, 389.2785) (-140.4847, 389.3279) (-140.586, 389.3551) knots 0 0 0 1 2 2 2
  spline S183 degree 2 poles (-140.586, 389.3551) (-140.8478, 389.4317) (-141.0849, 389.7478) (-141.0849, 389.9726) knots 0 0 0 1 2 2 2
  spline S184 degree 2 poles (-141.0849, 389.9726) (-141.0849, 390.2838) (-140.6181, 390.6716) (-140.2328, 390.6716) knots 0 0 0 1 2 2 2
  spline S185 degree 2 poles (-140.2328, 390.6716) (-140.0426, 390.6716) (-139.6572, 390.5778) (-139.5263, 390.5061) knots 0 0 0 1 2 2 2
  line L133 (-139.5263, 390.5061) -> (-139.5263, 390.0936)
  line L134 (-139.5263, 390.0936) -> (-139.5461, 390.0936)
  spline S186 degree 2 poles (-139.5461, 390.0936) (-139.6943, 390.2122) (-140.0549, 390.348) (-140.2402, 390.348) knots 0 0 0 1 2 2 2
  spline S187 degree 2 poles (-140.2402, 390.348) (-140.4304, 390.348) (-140.6922, 390.1875) (-140.6922, 390.0269) knots 0 0 0 1 2 2 2
  spline S188 degree 2 poles (-140.6922, 390.0269) (-140.6922, 389.8812) (-140.5366, 389.7404) (-140.3637, 389.696) knots 0 0 0 1 2 2 2
  spline S189 degree 2 poles (-140.3637, 389.696) (-140.2797, 389.6737) (-140.0673, 389.6293) (-139.9512, 389.6021) knots 0 0 0 1 2 2 2
  spline S190 degree 2 poles (-139.9512, 389.6021) (-139.6992, 389.5379) (-139.4424, 389.2439) (-139.4424, 388.9895) knots 0 0 0 1 2 2 2
  spline S191 degree 2 poles (-139.4424, 388.9895) (-139.4424, 388.8413) (-139.5584, 388.5795) (-139.6721, 388.4832) knots 0 0 0 1 2 2 2
  spline S192 degree 2 poles (-139.6721, 388.4832) (-139.7931, 388.3819) (-140.1019, 388.2757) (-140.3365, 388.2757) knots 0 0 0 1 2 2 2
  spline S193 degree 2 poles (-138.3926, 388.2856) (-138.7063, 388.2856) (-139.0595, 388.6437) (-139.0595, 389.0315) knots 0 0 0 1 2 2 2
  line L135 (-139.0595, 389.0315) -> (-139.0595, 390.2986)
  line L136 (-139.0595, 390.2986) -> (-139.3189, 390.2986)
  line L137 (-139.3189, 390.2986) -> (-139.3189, 390.6173)
  line L138 (-139.3189, 390.6173) -> (-139.0595, 390.6173)
  line L139 (-139.0595, 390.6173) -> (-139.0595, 391.2743)
  line L140 (-139.0595, 391.2743) -> (-138.6742, 391.2743)
  line L141 (-138.6742, 391.2743) -> (-138.6742, 390.6173)
  line L142 (-138.6742, 390.6173) -> (-137.9653, 390.6173)
  line L143 (-137.9653, 390.6173) -> (-137.9653, 390.2986)
  line L144 (-137.9653, 390.2986) -> (-138.6742, 390.2986)
  line L145 (-138.6742, 390.2986) -> (-138.6742, 389.2094)
  spline S194 degree 2 poles (-138.6742, 389.2094) (-138.6742, 389.0365) (-138.6618, 388.8463) (-138.6198, 388.7648) knots 0 0 0 1 2 2 2
  spline S195 degree 2 poles (-138.6198, 388.7648) (-138.5853, 388.6931) (-138.4297, 388.6215) (-138.2963, 388.6215) knots 0 0 0 1 2 2 2
  spline S196 degree 2 poles (-138.2963, 388.6215) (-138.2024, 388.6215) (-138.027, 388.6783) (-137.9875, 388.6956) knots 0 0 0 1 2 2 2
  line L146 (-137.9875, 388.6956) -> (-137.9653, 388.6956)
  line L147 (-137.9653, 388.6956) -> (-137.9653, 388.3498)
  spline S197 degree 2 poles (-137.9653, 388.3498) (-138.074, 388.3202) (-138.2963, 388.2856) (-138.3926, 388.2856) knots 0 0 0 1 2 2 2
  line L148 (-137.2885, 388.33) -> (-137.6738, 388.33)
  line L149 (-137.6738, 388.33) -> (-137.6738, 390.6173)
  line L150 (-137.6738, 390.6173) -> (-137.2885, 390.6173)
  line L151 (-137.2885, 390.6173) -> (-137.2885, 388.33)
  line L152 (-137.2613, 390.9977) -> (-137.6985, 390.9977)
  line L153 (-137.6985, 390.9977) -> (-137.6985, 391.3978)
  line L154 (-137.6985, 391.3978) -> (-137.2613, 391.3978)
  line L155 (-137.2613, 391.3978) -> (-137.2613, 390.9977)
  spline S198 degree 2 poles (-135.8139, 388.2782) (-136.051, 388.2782) (-136.4438, 388.4239) (-136.5845, 388.5721) knots 0 0 0 1 2 2 2
  spline S199 degree 2 poles (-136.5845, 388.5721) (-136.7253, 388.7178) (-136.881, 389.1674) (-136.881, 389.4687) knots 0 0 0 1 2 2 2
  spline S200 degree 2 poles (-136.881, 389.4687) (-136.881, 389.7701) (-136.7204, 390.2097) (-136.5845, 390.3579) knots 0 0 0 1 2 2 2
  spline S201 degree 2 poles (-136.5845, 390.3579) (-136.4487, 390.5086) (-136.0461, 390.6691) (-135.8139, 390.6691) knots 0 0 0 1 2 2 2
  spline S202 degree 2 poles (-135.8139, 390.6691) (-135.6262, 390.6691) (-135.2754, 390.5629) (-135.1396, 390.4938) knots 0 0 0 1 2 2 2
  line L156 (-135.1396, 390.4938) -> (-135.1396, 390.0615)
  line L157 (-135.1396, 390.0615) -> (-135.1618, 390.0615)
  spline S203 degree 2 poles (-135.1618, 390.0615) (-135.2038, 390.0961) (-135.3323, 390.185) (-135.4236, 390.232) knots 0 0 0 1 2 2 2
  spline S204 degree 2 poles (-135.4236, 390.232) (-135.5052, 390.2715) (-135.7225, 390.3332) (-135.8213, 390.3332) knots 0 0 0 1 2 2 2
  spline S205 degree 2 poles (-135.8213, 390.3332) (-136.1202, 390.3332) (-136.4833, 389.8812) (-136.4833, 389.4687) knots 0 0 0 1 2 2 2
  spline S206 degree 2 poles (-136.4833, 389.4687) (-136.4833, 389.0661) (-136.1325, 388.6141) (-135.8213, 388.6141) knots 0 0 0 1 2 2 2
  spline S207 degree 2 poles (-135.8213, 388.6141) (-135.6336, 388.6141) (-135.2927, 388.7697) (-135.1618, 388.8907) knots 0 0 0 1 2 2 2
  line L158 (-135.1618, 388.8907) -> (-135.1396, 388.8907)
  line L159 (-135.1396, 388.8907) -> (-135.1396, 388.4585)
  spline S208 degree 2 poles (-135.1396, 388.4585) (-135.1964, 388.4313) (-135.3693, 388.3547) (-135.4385, 388.3375) knots 0 0 0 1 2 2 2
  spline S209 degree 2 poles (-135.4385, 388.3375) (-135.5373, 388.3078) (-135.6929, 388.2782) (-135.8139, 388.2782) knots 0 0 0 1 2 2 2
  line L160 (-132.8943, 388.33) -> (-133.4007, 388.33)
  line L161 (-133.4007, 388.33) -> (-134.2504, 389.4341)
  line L162 (-134.2504, 389.4341) -> (-134.4035, 389.2859)
  line L163 (-134.4035, 389.2859) -> (-134.4035, 388.33)
  line L164 (-134.4035, 388.33) -> (-134.7888, 388.33)
  line L165 (-134.7888, 388.33) -> (-134.7888, 391.5139)
  line L166 (-134.7888, 391.5139) -> (-134.4035, 391.5139)
  line L167 (-134.4035, 391.5139) -> (-134.4035, 389.6515)
  line L168 (-134.4035, 389.6515) -> (-133.4995, 390.6173)
  line L169 (-133.4995, 390.6173) -> (-133.0203, 390.6173)
  line L170 (-133.0203, 390.6173) -> (-133.9589, 389.6614)
  line L171 (-133.9589, 389.6614) -> (-132.8943, 388.33)
  spline S210 degree 2 poles (-132.0842, 388.2757) (-132.3139, 388.2757) (-132.7116, 388.3992) (-132.8425, 388.4684) knots 0 0 0 1 2 2 2
  line L172 (-132.8425, 388.4684) -> (-132.8425, 388.9006)
  line L173 (-132.8425, 388.9006) -> (-132.8227, 388.9006)
  spline S211 degree 2 poles (-132.8227, 388.9006) (-132.7733, 388.8611) (-132.6399, 388.7672) (-132.5288, 388.7154) knots 0 0 0 1 2 2 2
  spline S212 degree 2 poles (-132.5288, 388.7154) (-132.4325, 388.6684) (-132.1953, 388.5993) (-132.0694, 388.5993) knots 0 0 0 1 2 2 2
  spline S213 degree 2 poles (-132.0694, 388.5993) (-131.978, 388.5993) (-131.768, 388.6413) (-131.7186, 388.6758) knots 0 0 0 1 2 2 2
  spline S214 degree 2 poles (-131.7186, 388.6758) (-131.647, 388.7228) (-131.5828, 388.829) (-131.5828, 388.9377) knots 0 0 0 1 2 2 2
  spline S215 degree 2 poles (-131.5828, 388.9377) (-131.5828, 389.0735) (-131.731, 389.2143) (-131.9212, 389.2612) knots 0 0 0 1 2 2 2
  spline S216 degree 2 poles (-131.9212, 389.2612) (-131.9953, 389.2785) (-132.2324, 389.3279) (-132.3337, 389.3551) knots 0 0 0 1 2 2 2
  spline S217 degree 2 poles (-132.3337, 389.3551) (-132.5955, 389.4317) (-132.8326, 389.7478) (-132.8326, 389.9726) knots 0 0 0 1 2 2 2
  spline S218 degree 2 poles (-132.8326, 389.9726) (-132.8326, 390.2838) (-132.3658, 390.6716) (-131.9804, 390.6716) knots 0 0 0 1 2 2 2
  spline S219 degree 2 poles (-131.9804, 390.6716) (-131.7902, 390.6716) (-131.4049, 390.5778) (-131.274, 390.5061) knots 0 0 0 1 2 2 2
  line L174 (-131.274, 390.5061) -> (-131.274, 390.0936)
  line L175 (-131.274, 390.0936) -> (-131.2938, 390.0936)
  spline S220 degree 2 poles (-131.2938, 390.0936) (-131.442, 390.2122) (-131.8026, 390.348) (-131.9878, 390.348) knots 0 0 0 1 2 2 2
  spline S221 degree 2 poles (-131.9878, 390.348) (-132.178, 390.348) (-132.4399, 390.1875) (-132.4399, 390.0269) knots 0 0 0 1 2 2 2
  spline S222 degree 2 poles (-132.4399, 390.0269) (-132.4399, 389.8812) (-132.2843, 389.7404) (-132.1113, 389.696) knots 0 0 0 1 2 2 2
  spline S223 degree 2 poles (-132.1113, 389.696) (-132.0274, 389.6737) (-131.8149, 389.6293) (-131.6989, 389.6021) knots 0 0 0 1 2 2 2
  spline S224 degree 2 poles (-131.6989, 389.6021) (-131.4469, 389.5379) (-131.19, 389.2439) (-131.19, 388.9895) knots 0 0 0 1 2 2 2
  spline S225 degree 2 poles (-131.19, 388.9895) (-131.19, 388.8413) (-131.3061, 388.5795) (-131.4197, 388.4832) knots 0 0 0 1 2 2 2
  spline S226 degree 2 poles (-131.4197, 388.4832) (-131.5408, 388.3819) (-131.8495, 388.2757) (-132.0842, 388.2757) knots 0 0 0 1 2 2 2
  spline S227 degree 2 poles (-127.6431, 389.4737) (-127.6431, 388.8957) (-128.1988, 388.2658) (-128.6632, 388.2658) knots 0 0 0 1 2 2 2
  spline S228 degree 2 poles (-128.6632, 388.2658) (-129.1399, 388.2658) (-129.6858, 388.9154) (-129.6858, 389.4737) knots 0 0 0 1 2 2 2
  spline S229 degree 2 poles (-129.6858, 389.4737) (-129.6858, 390.0467) (-129.1226, 390.6815) (-128.6632, 390.6815) knots 0 0 0 1 2 2 2
  spline S230 degree 2 poles (-128.6632, 390.6815) (-128.1988, 390.6815) (-127.6431, 390.0492) (-127.6431, 389.4737) knots 0 0 0 1 2 2 2
  spline S231 degree 2 poles (-128.0408, 389.4737) (-128.0408, 389.9183) (-128.3643, 390.3505) (-128.6632, 390.3505) knots 0 0 0 1 2 2 2
  spline S232 degree 2 poles (-128.6632, 390.3505) (-128.9621, 390.3505) (-129.2881, 389.9183) (-129.2881, 389.4737) knots 0 0 0 1 2 2 2
  spline S233 degree 2 poles (-129.2881, 389.4737) (-129.2881, 389.0414) (-128.9621, 388.5968) (-128.6632, 388.5968) knots 0 0 0 1 2 2 2
  spline S234 degree 2 poles (-128.6632, 388.5968) (-128.3668, 388.5968) (-128.0408, 389.034) (-128.0408, 389.4737) knots 0 0 0 1 2 2 2
  line L176 (-126.0351, 390.2048) -> (-126.0549, 390.2048)
  spline S235 degree 2 poles (-126.0549, 390.2048) (-126.0993, 390.2171) (-126.1957, 390.2221) (-126.2624, 390.2221) knots 0 0 0 1 2 2 2
  spline S236 degree 2 poles (-126.2624, 390.2221) (-126.418, 390.2221) (-126.7242, 390.0862) (-126.8626, 389.9528) knots 0 0 0 1 2 2 2
  line L177 (-126.8626, 389.9528) -> (-126.8626, 388.33)
  line L178 (-126.8626, 388.33) -> (-127.2479, 388.33)
  line L179 (-127.2479, 388.33) -> (-127.2479, 390.6173)
  line L180 (-127.2479, 390.6173) -> (-126.8626, 390.6173)
  line L181 (-126.8626, 390.6173) -> (-126.8626, 390.2764)
  spline S237 degree 2 poles (-126.8626, 390.2764) (-126.6526, 390.4641) (-126.3389, 390.6173) (-126.1907, 390.6173) knots 0 0 0 1 2 2 2
  spline S238 degree 2 poles (-126.1907, 390.6173) (-126.1314, 390.6173) (-126.0722, 390.6123) (-126.0351, 390.6049) knots 0 0 0 1 2 2 2
  line L182 (-126.0351, 390.6049) -> (-126.0351, 390.2048)
  line L183 (-121.6558, 390.6173) -> (-122.2362, 388.33)
  line L184 (-122.2362, 388.33) -> (-122.5919, 388.33)
  line L185 (-122.5919, 388.33) -> (-123.1501, 390.0936)
  line L186 (-123.1501, 390.0936) -> (-123.7059, 388.33)
  line L187 (-123.7059, 388.33) -> (-124.0591, 388.33)
  line L188 (-124.0591, 388.33) -> (-124.6445, 390.6173)
  line L189 (-124.6445, 390.6173) -> (-124.2443, 390.6173)
  line L190 (-124.2443, 390.6173) -> (-123.8393, 388.8463)
  line L191 (-123.8393, 388.8463) -> (-123.2983, 390.6173)
  line L192 (-123.2983, 390.6173) -> (-122.9797, 390.6173)
  line L193 (-122.9797, 390.6173) -> (-122.4239, 388.8463)
  line L194 (-122.4239, 388.8463) -> (-122.0436, 390.6173)
  line L195 (-122.0436, 390.6173) -> (-121.6558, 390.6173)
  line L196 (-119.5217, 388.33) -> (-119.907, 388.33)
  line L197 (-119.907, 388.33) -> (-119.907, 389.6342)
  spline S239 degree 2 poles (-119.907, 389.6342) (-119.907, 389.7923) (-119.9366, 390.064) (-119.9811, 390.1455) knots 0 0 0 1 2 2 2
  spline S240 degree 2 poles (-119.9811, 390.1455) (-120.028, 390.232) (-120.196, 390.3159) (-120.3393, 390.3159) knots 0 0 0 1 2 2 2
  spline S241 degree 2 poles (-120.3393, 390.3159) (-120.4825, 390.3159) (-120.7863, 390.1628) (-120.9321, 390.0393) knots 0 0 0 1 2 2 2
  line L198 (-120.9321, 390.0393) -> (-120.9321, 388.33)
  line L199 (-120.9321, 388.33) -> (-121.3174, 388.33)
  line L200 (-121.3174, 388.33) -> (-121.3174, 391.5139)
  line L201 (-121.3174, 391.5139) -> (-120.9321, 391.5139)
  line L202 (-120.9321, 391.5139) -> (-120.9321, 390.3629)
  spline S242 degree 2 poles (-120.9321, 390.3629) (-120.7592, 390.5185) (-120.4257, 390.6815) (-120.238, 390.6815) knots 0 0 0 1 2 2 2
  spline S243 degree 2 poles (-120.238, 390.6815) (-119.9021, 390.6815) (-119.5217, 390.2369) (-119.5217, 389.8145) knots 0 0 0 1 2 2 2
  line L203 (-119.5217, 389.8145) -> (-119.5217, 388.33)
  spline S244 degree 2 poles (-117.7062, 388.5721) (-117.7531, 388.5375) (-117.9112, 388.414) (-117.9853, 388.377) knots 0 0 0 1 2 2 2
  spline S245 degree 2 poles (-117.9853, 388.377) (-118.0866, 388.3226) (-118.2768, 388.2658) (-118.4497, 388.2658) knots 0 0 0 1 2 2 2
  spline S246 degree 2 poles (-118.4497, 388.2658) (-118.5905, 388.2658) (-118.8449, 388.372) (-118.9412, 388.4684) knots 0 0 0 1 2 2 2
  spline S247 degree 2 poles (-118.9412, 388.4684) (-119.0326, 388.5622) (-119.1438, 388.8389) (-119.1438, 388.992) knots 0 0 0 1 2 2 2
  spline S248 degree 2 poles (-119.1438, 388.992) (-119.1438, 389.2291) (-118.9437, 389.5651) (-118.7263, 389.6614) knots 0 0 0 1 2 2 2
  spline S249 degree 2 poles (-118.7263, 389.6614) (-118.5337, 389.7503) (-118.01, 389.817) (-117.7062, 389.8343) knots 0 0 0 1 2 2 2
  line L204 (-117.7062, 389.8343) -> (-117.7062, 389.9084)
  spline S250 degree 2 poles (-117.7062, 389.9084) (-117.7062, 390.0418) (-117.7877, 390.2073) (-117.8618, 390.2542) knots 0 0 0 1 2 2 2
  spline S251 degree 2 poles (-117.8618, 390.2542) (-117.9359, 390.3011) (-118.1483, 390.3308) (-118.262, 390.3308) knots 0 0 0 1 2 2 2
  spline S252 degree 2 poles (-118.262, 390.3308) (-118.3953, 390.3308) (-118.756, 390.2517) (-118.9363, 390.1751) knots 0 0 0 1 2 2 2
  line L205 (-118.9363, 390.1751) -> (-118.9585, 390.1751)
  line L206 (-118.9585, 390.1751) -> (-118.9585, 390.5679)
  spline S253 degree 2 poles (-118.9585, 390.5679) (-118.8523, 390.5975) (-118.4546, 390.6716) (-118.2595, 390.6716) knots 0 0 0 1 2 2 2
  spline S254 degree 2 poles (-118.2595, 390.6716) (-118.0224, 390.6716) (-117.6988, 390.5975) (-117.5704, 390.5012) knots 0 0 0 1 2 2 2
  spline S255 degree 2 poles (-117.5704, 390.5012) (-117.4444, 390.4073) (-117.3209, 390.1085) (-117.3209, 389.8936) knots 0 0 0 1 2 2 2
  line L207 (-117.3209, 389.8936) -> (-117.3209, 388.33)
  line L208 (-117.3209, 388.33) -> (-117.7062, 388.33)
  line L209 (-117.7062, 388.33) -> (-117.7062, 388.5721)
  line L210 (-117.7062, 388.8932) -> (-117.7062, 389.528)
  spline S256 degree 2 poles (-117.7062, 389.528) (-117.8445, 389.5157) (-118.262, 389.4737) (-118.3929, 389.4341) knots 0 0 0 1 2 2 2